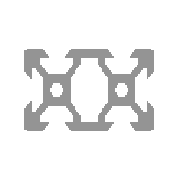
# Autodesk Inventor part: vslot 20 x 40
Saved by Autodesk Inventor 2015 (Build 190159000, 159)
## iProperties
Created: 2013-06-18
Part Number: vslot 20 x 40
Material: Aluminum 6061
Document SubType Name: Modeling
Designer: Jon Hollander
Density: 2.71 g/cm^3
Categories: <MemberInstance><Categories><Category DisplayName="Structural Shapes" InternalName="089c4875-fa83-4c05-b084-43b9cc11f5ed" Mnemonic="GRDR"><CategoryParameter DisplayName="Custom Base Point" InternalName="4f1d1b73-316d-484b-a3df-9cbabb16eb77" Mnemonic="shpBasePoint"/><CategoryParameter DisplayName="FG Authored" InternalName="9c666724-f362-4ea7-ac62-f6a007de5c69" Mnemonic="shpFGAuto"/><CategoryParameter DisplayName="Legacy Member ID" InternalName="340afe4f-75d7-48d3-ab7d-943f3c3da468" Mnemonic="LegacyMemberID"/><CategoryParameter DisplayName="Base Length" InternalName="42e34263-8f20-4d0e-ad48-bf1385b87c24" Mnemonic="shplen"/><CategoryParameter DisplayName="Distance of the Center of Gravity X-X" InternalName="26c9bdb8-9c79-4b4f-a92e-8e197583c9c4" Mnemonic="grcendistX"/><CategoryParameter DisplayName="Distance of the Center of Gravity Y-Y" InternalName="bcc4fb17-7af4-436a-8f8c-d0aa3b0248c5" Mnemonic="grcendistY"/><CategoryParameter DisplayName="Torsional Rigidity Modulus" InternalName="26c1ec35-5026-4c63-ad0a-751cf684a536" Mnemonic="torrigmod"/><CategoryParameter DisplayName="Torsional Section Modulus" InternalName="7c55a8dc-8844-49f9-a867-cc677b30ec9a" Mnemonic="torsecmod"/><CategoryParameter DisplayName="Coefficient of Shear Displacement" InternalName="de4c90c6-aaa8-468f-a335-6737b311b5d3" Mnemonic="shdispc"/><CategoryParameter DisplayName="Section Area" InternalName="1ff91680-64b0-4202-b9a3-7fd3f94bba3b" Mnemonic="secarea"/><CategoryParameter DisplayName="Moment of Inertia (x)" InternalName="4cd780bc-73d7-43ac-917a-579e5cbd684d" Mnemonic="inermomx"/><CategoryParameter DisplayName="Moment of Inertia (y)" InternalName="4b9f58ea-bced-460e-81ea-3d29ca5a49e3" Mnemonic="inermomy"/><CategoryParameter DisplayName="Section Module (x)" InternalName="72cfad18-cf51-4ed4-aaa7-c6b224f8419f" Mnemonic="secmodx"/><CategoryParameter DisplayName="Section Module (y)" InternalName="59eaa5e9-d227-48dc-b6c1-6920f96e0f95" Mnemonic="secmody"/><CategoryParameter DisplayName="Radius of Gyration (x)" InternalName="25778675-03e9-40c1-b6a8-4a9ed693320d" Mnemonic="gyrradx"/><CategoryParameter DisplayName="Radius of Gyration (y)" InternalName="bfa18ebe-1636-4dbe-8d42-b263e0b73184" Mnemonic="gyrrady"/><CategoryParameter DisplayName="Shape Thickness" InternalName="d109cf76-8eb4-42fc-9800-4409734adc67" Mnemonic="shpthick"/><CategoryParameter DisplayName="Second Shape Thickness" InternalName="9251a8e1-85fd-4e47-af99-afdb762317d9" Mnemonic="shpthick2"/><CategoryParameter DisplayName="Shape Width" InternalName="7c717d54-a18f-4666-b4d4-573cce22c62c" Mnemonic="shpwdth"/><CategoryParameter DisplayName="Shape Height" InternalName="50274e7d-5ac0-4796-92cb-c59e54983c67" Mnemonic="shpheig"/><CategoryParameter DisplayName="Mass per Length Unit" InternalName="0bb95a10-148f-4027-a459-38d7b056702a" Mnemonic="shpmass"/><CategoryParameter DisplayName="Section Designation" InternalName="5a64d034-428d-49c8-ba32-7619764de20f" Mnemonic="shpdes"/><Category DisplayName="Square/Rectangular Tubes" InternalName="afc8e2d8-05d6-4609-8807-f98a9b7d2ed0" Mnemonic="SQRSHP"><CategoryParameter DisplayName="Moment of Inertia (x)" InternalName="8c4637b6-6b69-4878-9d5d-26a32185d655" Mnemonic="inermomx"/><CategoryParameter DisplayName="Moment of Inertia (y)" InternalName="55ec8510-8276-4c45-8f10-594e0fee7eb3" Mnemonic="inermomy"/><CategoryParameter DisplayName="Section Module (x)" InternalName="50d965a6-04bf-46b9-8ace-861858d348e6" Mnemonic="secmodx"/><CategoryParameter DisplayName="Section Module (y)" InternalName="5106aeac-54a2-4159-a9af-8933dd39dba2" Mnemonic="secmody"/><CategoryParameter DisplayName="Section Area" InternalName="2f7f79dd-983c-4263-802a-5b6a1495fdc5" Mnemonic="secarea"/><CategoryParameter DisplayName="Radius of Gyration (x)" InternalName="56c89926-a299-4389-a862-ac94c9691272" Mnemonic="gyrradx"/><CategoryParameter DisplayName="Radius of Gyration (y)" InternalName="fa48a7f5-f030-40f9-a60b-de8a845b7104" Mnemonic="gyrrady"/><CategoryParameter DisplayName="Shape Width" InternalName="8c8a1782-5e80-4d77-858b-304b1c0ad1fd" Mnemonic="shpwdth"/><CategoryParameter DisplayName="Shape Thickness" InternalName="52712fc5-f4ee-4eda-b3f2-6fce82c26419" Mnemonic="shpthick"/><CategoryParameter DisplayName="Radius" InternalName="5d8d062c-e28e-41c1-98da-8e5fee36da1a" Mnemonic="shprad"/></Category></Category></Categories><FamilyTemplate Id="vslot 20 x 40"><FamilyTemplateParameters><FamilyTemplateParameter ObjectType="kModelParameterObject" ValueType="xs:double" Id="12" ObjectReferenceKey="Length"/></FamilyTemplateParameters></FamilyTemplate><CategoryParameterMap><ParamToTemplateMap><ParamToTemplate CategoryParameter="//CategoryParameter[@InternalName='42e34263-8f20-4d0e-ad48-bf1385b87c24']" TemplateParameter="12"/><ParamToTemplate CategoryParameter="//CategoryParameter[@InternalName='9c666724-f362-4ea7-ac62-f6a007de5c69']" ConstantValue="1"/></ParamToTemplateMap></CategoryParameterMap></MemberInstance>
Mass: 100.661 g
Surface Area: 378.692 cm^2
Volume: 37.1442 cm^3
Appearance: Aluminum - Flat
G_L: 10.000 mm
Author: Jon Hollander
Autodesk Inventor part; units mm, degrees
ref_plane "YZ Plane" through (0, 0, 0) normal (1, 0, 0) x (0, 1, 0)
ref_plane "XZ Plane" through (0, 0, 0) normal (0, 1, 0) x (-1, 0, 0)
ref_plane "Start Plane" through (0, 0, 0) normal (0, 0, 1) x (1, 0, 0)
ref_plane "End Plane" through (0, 0, 10) normal (0, 0, 1) x (1, 0, 0)
sketch "Sketch3" plane through (0, 0, 0) normal (0, 0, 1) x (1, 0, 0)
  line L0 (0, 0) -> (0, 10) construction
  line L1 (-10, 10) -> (-10, 0) construction
  line L2 (0, 0) -> (-10, 0) construction
  circle A0 centre (-10, 0) radius 2.1
  line L3 (-13.9007, 3.9007) -> (-6.0993, 3.9007) construction
  line L4 (-6.0993, 3.9007) -> (-6.0993, -3.9007) construction
  line L5 (-6.0993, -3.9007) -> (-13.9007, -3.9007) construction
  line L6 (-13.9007, -3.9007) -> (-13.9007, 3.9007) construction
  line L7 (-13.9007, 3.9007) -> (-6.0993, -3.9007) construction
  line L8 (-6.0993, 3.9007) -> (-13.9007, -3.9007) construction
  line L9 (-13.9007, -2.84) -> (-12.84, -3.9007) construction
  line L10 (-13.9007, -2.84) -> (-12.4007, -2.84) construction
  line L11 (-12.84, -3.9007) -> (-15.4993, -6.56)
  line L12 (-15.4993, -6.56) -> (-15.4993, -8.2)
  line L13 (-15.4993, -8.2) -> (-12.84, -8.2)
  line L14 (-12.84, -8.2) -> (-14.64, -10)
  line L15 (-7.16, -3.9007) -> (-4.5007, -6.56)
  line L16 (-4.5007, -6.56) -> (-4.5007, -8.2)
  line L17 (-4.5007, -8.2) -> (-7.16, -8.2)
  line L18 (-7.16, -8.2) -> (-5.36, -10)
  line L19 (-12.84, -3.9007) -> (-7.16, -3.9007)
  line L20 (-12.84, 3.9007) -> (-13.9007, 2.84) construction
  line L21 (-12.84, 3.9007) -> (-12.84, 2.4007) construction
  line L22 (-13.9007, 2.84) -> (-16.56, 5.4993)
  line L23 (-16.56, 5.4993) -> (-18.2, 5.4993)
  line L24 (-18.2, 5.4993) -> (-18.2, 2.84)
  line L25 (-18.2, 2.84) -> (-20, 4.64)
  line L26 (-18.2, -2.84) -> (-20, -4.64)
  line L27 (-18.2, -5.4993) -> (-18.2, -2.84)
  line L28 (-16.56, -5.4993) -> (-18.2, -5.4993)
  line L29 (-13.9007, -2.84) -> (-16.56, -5.4993)
  line L30 (-13.9007, 2.84) -> (-13.9007, -2.84)
  line L31 (-6.0993, 2.84) -> (-7.16, 3.9007) construction
  line L32 (-6.0993, 2.84) -> (-7.5993, 2.84) construction
  line L33 (-7.16, 3.9007) -> (-4.5007, 6.56)
  line L34 (-4.5007, 6.56) -> (-4.5007, 8.2)
  line L35 (-4.5007, 8.2) -> (-7.16, 8.2)
  line L36 (-7.16, 8.2) -> (-5.36, 10)
  line L37 (-12.84, 8.2) -> (-14.64, 10)
  line L38 (-15.4993, 8.2) -> (-12.84, 8.2)
  line L39 (-15.4993, 6.56) -> (-15.4993, 8.2)
  line L40 (-12.84, 3.9007) -> (-15.4993, 6.56)
  line L41 (-7.16, 3.9007) -> (-12.84, 3.9007)
  line L42 (-6.0993, 2.84) -> (-2.6993, 6.24)
  line L43 (-2.6993, 6.24) -> (-2.6993, 8.2)
  line L44 (-4.5007, 8.2) -> (0, 8.2) construction
  line L45 (-6.0993, -2.84) -> (-2.6993, -6.24)
  line L46 (-2.6993, -6.24) -> (-2.6993, -8.2)
  line L47 (10, 10) -> (10, 0) construction
  circle A1 centre (10, 0) radius 2.1
  line L48 (13.9007, 3.9007) -> (6.0993, -3.9007) construction
  line L49 (13.9007, -2.84) -> (12.84, -3.9007) construction
  line L50 (12.84, -3.9007) -> (15.4993, -6.56)
  line L51 (15.4993, -6.56) -> (15.4993, -8.2)
  line L52 (15.4993, -8.2) -> (12.84, -8.2)
  line L53 (12.84, -8.2) -> (14.64, -10)
  line L54 (7.16, -8.2) -> (5.36, -10)
  line L55 (4.5007, -8.2) -> (7.16, -8.2)
  line L56 (4.5007, -6.56) -> (4.5007, -8.2)
  line L57 (7.16, -3.9007) -> (4.5007, -6.56)
  line L58 (12.84, -3.9007) -> (7.16, -3.9007)
  line L59 (13.9007, 2.84) -> (13.9007, -2.84)
  line L60 (13.9007, 2.84) -> (16.56, 5.4993)
  line L61 (16.56, 5.4993) -> (18.2, 5.4993)
  line L62 (18.2, 5.4993) -> (18.2, 2.84)
  line L63 (18.2, 2.84) -> (20, 4.64)
  line L64 (18.2, -5.4993) -> (18.2, -2.84)
  line L65 (18.2, -2.84) -> (20, -4.64)
  line L66 (16.56, -5.4993) -> (18.2, -5.4993)
  line L67 (13.9007, -2.84) -> (16.56, -5.4993)
  line L68 (7.16, 3.9007) -> (12.84, 3.9007)
  line L69 (7.16, 3.9007) -> (4.5007, 6.56)
  line L70 (4.5007, 6.56) -> (4.5007, 8.2)
  line L71 (4.5007, 8.2) -> (7.16, 8.2)
  line L72 (7.16, 8.2) -> (5.36, 10)
  line L73 (15.4993, 8.2) -> (12.84, 8.2)
  line L74 (12.84, 8.2) -> (14.64, 10)
  line L75 (15.4993, 6.56) -> (15.4993, 8.2)
  line L76 (12.84, 3.9007) -> (15.4993, 6.56)
  line L77 (6.0993, 2.84) -> (2.6993, 6.24)
  line L78 (2.6993, 6.24) -> (2.6993, 8.2)
  line L79 (6.0993, -2.84) -> (2.6993, -6.24)
  line L80 (2.6993, -6.24) -> (2.6993, -8.2)
  line L81 (-14.64, -10) -> (-18.2, -10)
  line L82 (-20, -8.2) -> (-20, -4.64)
  line L83 (-20, 4.64) -> (-20, 8.2)
  line L84 (-18.2, 10) -> (-14.64, 10)
  line L85 (18.2, -10) -> (14.64, -10)
  line L86 (5.36, -10) -> (-5.36, -10)
  line L87 (-5.36, 10) -> (5.36, 10)
  line L88 (14.64, 10) -> (18.2, 10)
  line L89 (20, 8.2) -> (20, 4.64)
  line L90 (20, -4.64) -> (20, -8.2)
  line L91 (-2.6993, -8.2) -> (2.6993, -8.2)
  line L92 (-2.6993, 8.2) -> (2.6993, 8.2)
  line L93 (-6.0993, 2.84) -> (-6.0993, -2.84)
  line L94 (6.0993, 2.84) -> (6.0993, -2.84)
  arc A2 (-20, -8.2) -> (-18.2, -10) centre (-18.2, -8.2) ccw
  arc A3 (-18.2, 10) -> (-20, 8.2) centre (-18.2, 8.2) ccw
  arc A4 (18.2, -10) -> (20, -8.2) centre (18.2, -8.2) ccw
  arc A5 (20, 8.2) -> (18.2, 10) centre (18.2, 8.2) ccw
  point P0 (-13.9007, -3.9007)
  point P1 (-13.9007, 3.9007)
  point P2 (-13.9007, 3.9007)
  point P3 (-6.0993, 3.9007)
  point P4 (6.0993, 3.9007)
  point P5 (13.9007, -3.9007)
  point P6 (12.4007, -2.84)
  point P7 (13.9007, -3.9007)
  point P8 (13.9007, 3.9007)
  point P9 (12.84, 3.9007)
  point P10 (12.84, 2.4007)
  point P11 (13.9007, 3.9007)
  point P12 (6.0993, 3.9007)
  point P13 (7.5993, 2.84)
  point P14 (-20, 10)
  point P15 (20, -10)
  point P16 (20, 10)
  point P17 (-20, -10)
  dimension "d26" = 10
  dimension "d27" = 10
  dimension "d28" = 4.2
  dimension "d29" = 1.5
  dimension "d30" = 45
  dimension "d32" = 45
  dimension "d33" = 1.64
  dimension "d34" = 1.8
  dimension "d35" = 10
  dimension "d36" = 5.68
  dimension "d39" = 180
  dimension "d41" = 1.96
  dimension "d42" = 5.68
  dimension "d45" = 1.8
  constraints: 190 end point, 60 symmetric about line, 20 parallel, 17 perpendicular, 12 point on line, 8 point on circle, 8 tangent, 6 centre point, 5 horizontal, 3 equal radius, 3 midpoint, 2 coincident, 1 equal length, 1 vertical, 52 other
  measures "d26" distance of L0.start L0.end
  measures "d27" distance between parallel lines of L0 L1
  measures "d28" diameter of A0
  measures "d29" distance of L9.start L9.end
  measures "d30" angle of L9 L10
  measures "d32" angle of L13 L14
  measures "d33" distance of L11.end L12.end
  measures "d34" horizontal distance of L13.end L14.end
  measures "d35" vertical distance of L1.end L14.end
  measures "d36" distance of L9.end L15.start
  measures "d41" distance of L42.end L43.end
  measures "d42" distance of L18.start L13.end
  measures "d45" radius of A2
extrude "Body" add sketch "Sketch3" along normal blind 125
sketch "Sketch4" plane through (0, 0, 0) normal (0, 0, 1) x (1, 0, 0)
  line L0 (0, 0) -> (10, 0)
ref_plane "Work Plane3" through (0, 0, 0) normal (0, -1, 0) x (1, 0, 0)
sketch "Sketch5" plane through (0, 0, 0) normal (0, -1, 0) x (1, 0, 0)
  line L0 (-2, 0) -> (12, 0)
  line L1 (-2, 10) -> (12, 10)
  dimension "d51" = 10
  measures "d51" distance between parallel lines of L0 L1
equation "\"d42\" = d36"
equation "\"G_OFFSET_START\" = 0"
equation "\"G_OFFSET_END\" = 0"
equation "\"G_L\" = d51"
body "Solid1"
